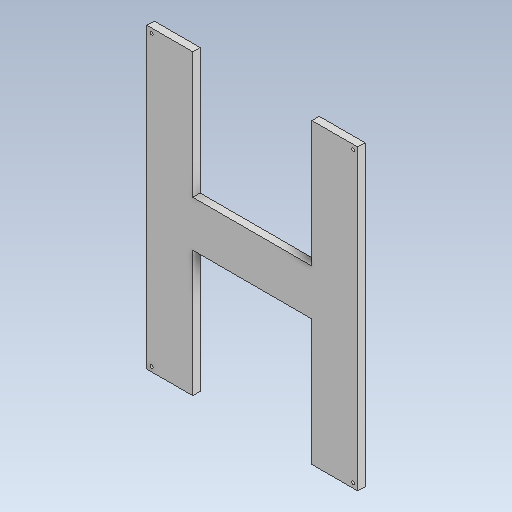
# Autodesk Inventor part: 0005-10-014 Suport Bed
Saved by Autodesk Inventor 2020 (Build 240168000, 168)
## iProperties
Created: 2020-12-19
Part Number: 0005-10-014 Suport Bed
Material: Generic
Document SubType Name: Modeling
Designer: Iulian Bors
Density: 1 g/cm^3
Appearance: Default
Author: Iulian Bors
Subject: 014
Autodesk Inventor part; units mm, degrees
ref_plane "YZ Plane" through (0, 0, 0) normal (1, 0, 0) x (0, 1, 0)
ref_plane "XZ Plane" through (0, 0, 0) normal (0, 1, 0) x (-1, 0, 0)
ref_plane "XY Plane" through (0, 0, 0) normal (0, 0, 1) x (1, 0, 0)
sketch "Sketch1" plane through (0, 0, 0) normal (0, 0, 1) x (1, 0, 0)
  line L0 (-115, 162.5) -> (115, 162.5)
  line L1 (115, 162.5) -> (115, -162.5)
  line L2 (115, -162.5) -> (-115, -162.5)
  line L3 (-115, -162.5) -> (-115, 162.5)
  point P0 (0, 0)
  point P1 (0, 162.5)
  point P2 (-115, 0)
  dimension "d0" = 230
  dimension "d1" = 325
  constraints: 8 end point, 2 midpoint, 2 parallel, 1 horizontal, 1 horizontal alignment, 1 perpendicular, 1 vertical alignment
  measures "d0" distance of L0.start L0.end
  measures "d1" distance of L0.end L1.end
extrude "Extrusion1" add sketch "Sketch1" along normal blind 8
sketch "Sketch2" plane through (0, 0, 8) normal (0, 0, 1) x (1, 0, 0)
  line L0 (-110, -157.5) -> (110, -157.5) construction
  line L1 (110, -157.5) -> (110, 157.5) construction
  line L2 (110, 157.5) -> (-110, 157.5) construction
  line L3 (-110, 157.5) -> (-110, -157.5) construction
  line L4 (-115, 162.5) -> (-115, -162.5) construction
  line L5 (115, 162.5) -> (-115, 162.5) construction
  point P0 (0, 0)
  point P1 (-110, 0)
  point P2 (-115, 0)
  point P3 (-115, 0)
  point P4 (0, 157.5)
  point P5 (0, 162.5)
  dimension "d4" = 5
  dimension "d5" = 5
  constraints: 8 end point, 5 midpoint, 4 coincident, 2 parallel, 1 horizontal, 1 horizontal alignment, 1 perpendicular, 1 vertical alignment
  measures "d4" distance between parallel lines of L4 L3
  measures "d5" distance between parallel lines of L5 L2
hole "Hole1" at (-110, -157.5, 8) at (-110, 157.5, 8) at (110, 157.5, 8) at (110, -157.5, 8) direction (0, 0, -1) diameter 3.5 end through all
sketch "Sketch3" plane through (0, 0, 8) normal (0, 0, 1) x (1, 0, 0)
  line L0 (65, -162.5) -> (-65, -162.5)
  line L1 (-65, -162.5) -> (-65, -25)
  line L2 (-65, -25) -> (65, -25)
  line L3 (65, -25) -> (65, -162.5)
  line L4 (-115, -162.5) -> (115, -162.5) projected
  line L5 (115, -162.5) -> (115, 162.5) projected
  line L6 (-115, 162.5) -> (-115, -162.5) projected
  line L7 (65, 25) -> (-65, 25)
  line L8 (-65, 25) -> (-65, 162.5)
  line L9 (-65, 162.5) -> (65, 162.5)
  line L10 (65, 162.5) -> (65, 25)
  line L11 (115, 162.5) -> (-115, 162.5) projected
  point P0 (0, 0)
  dimension "d13" = 50
  dimension "d14" = 50
  dimension "d15" = 25
  dimension "d16" = 25
  constraints: 16 end point, 4 collinear, 4 parallel, 2 horizontal, 2 perpendicular
  measures "d13" distance between parallel lines of L5 L3
  measures "d14" distance between parallel lines of L6 L1
  measures "d15" distance from line of point (0, 0) L2
  measures "d16" distance from line of point (0, 0) L7
extrude "Extrusion2" cut sketch "Sketch3" against normal blind 10 contours L0 L1 L2 L3 | L10 L7 L8 L9
body "Solid1"
